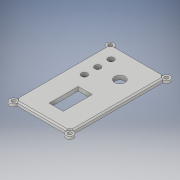
# Autodesk Inventor part: gora
Saved by Autodesk Inventor 2019 (Build 230136000, 136)
## iProperties
Created: 2019-09-16
Part Number: gora
Material: Ogólny
Document SubType Name: Modeling
Designer: mikol
Density: 1 g/cm^3
Appearance: Domyślna
Author: mikol
Autodesk Inventor part; units mm, degrees
ref_plane "YZ Plane" through (0, 0, 0) normal (1, 0, 0) x (0, 1, 0)
ref_plane "XZ Plane" through (0, 0, 0) normal (0, 1, 0) x (-1, 0, 0)
ref_plane "XY Plane" through (0, 0, 0) normal (0, 0, 1) x (1, 0, 0)
sketch "Sketch1" plane through (0, 0, 0) normal (0, 1, 0) x (-1, 0, 0)
  line L0 (32, 55) -> (-32, 55)
  line L1 (-32, 55) -> (-32, -55)
  line L2 (-32, -55) -> (32, -55)
  line L3 (32, -55) -> (32, 55)
  line L4 (32, 55) -> (-32, -55) construction
  line L5 (-32, 55) -> (32, -55) construction
  circle A0 centre (32, 55) radius 4.2425
  circle A1 centre (32, -55) radius 4.2425
  circle A2 centre (-32, 55) radius 4.2425
  circle A3 centre (-32, -55) radius 4.2425
  point P0 (0, 0)
  dimension "d0" = 64
  dimension "d1" = 110
  dimension "d2" = 8.485
  dimension "d5" = 110
  dimension "d8" = 64
  constraints: 12 end point, 4 centre point, 2 horizontal, 2 midpoint, 2 parallel, 1 coincident, 1 perpendicular, 1 vertical, 6 other
  measures "d0" distance of L2.end L1.end
  measures "d1" distance of L1.end L0.end
  measures "d2" diameter of A0
  measures "d5" distance of A0.centre A1.centre
  measures "d8" distance of A0.centre A2.centre
extrude "Extrusion1" add sketch "Sketch1" along normal blind 3
sketch "Sketch2" plane through (0, 3, 0) normal (0, 1, 0) x (1, 0, 0)
  line L0 (32, -50.7575) -> (32, 50.7575) projected
  arc A0 (32, 50.7575) -> (27.7575, 55) centre (32, 55) ccw projected
  line L1 (27.7575, 55) -> (-27.7575, 55) projected
  arc A1 (-27.7575, 55) -> (-32, 50.7575) centre (-32, 55) ccw projected
  line L2 (-32, 50.7575) -> (-32, -50.7575) projected
  arc A2 (-32, -50.7575) -> (-27.7575, -55) centre (-32, -55) ccw projected
  line L3 (-27.7575, -55) -> (27.7575, -55) projected
  arc A3 (27.7575, -55) -> (32, -50.7575) centre (32, -55) ccw projected
  circle A4 centre (-32, -55) radius 2.15
  circle A5 centre (-32, 55) radius 2.15
  circle A6 centre (32, -55) radius 2.15
  circle A7 centre (32, 55) radius 2.15
  point P0 (0, 0)
  dimension "d13" = 4.3
  dimension "d16" = 110
  dimension "d19" = 64
  constraints: 4 centre point, 1 coincident, 1 horizontal, 1 vertical, 6 other
  measures "d13" diameter of A4
  measures "d16" distance of A4.centre A5.centre
  measures "d19" distance of A4.centre A6.centre
extrude "Extrusion2" cut sketch "Sketch2" against normal blind 3 contours A4 | A5 | A6 | A7
sketch "Sketch3" plane through (0, 3, 0) normal (0, 1, 0) x (1, 0, 0)
  line L0 (-8, -38.5) -> (8, -38.5)
  line L1 (8, -38.5) -> (8, -5.5)
  line L2 (8, -5.5) -> (-8, -5.5)
  line L3 (-8, -5.5) -> (-8, -38.5)
  line L4 (-32, 50.7575) -> (-32, -50.7575) projected
  line L5 (32, -50.7575) -> (32, 50.7575) projected
  line L6 (-27.7575, -55) -> (27.7575, -55) projected
  point P0 (0, 0)
  dimension "d24" = 16
  dimension "d25" = 33
  dimension "d26" = 24
  dimension "d27" = 24
  dimension "d28" = 16.5
  constraints: 8 end point, 2 parallel, 1 horizontal, 1 perpendicular
  measures "d24" distance of L2.end L1.end
  measures "d25" distance of L1.end L0.end
  measures "d26" distance between parallel lines of L4 L3
  measures "d27" distance between parallel lines of L5 L1
  measures "d28" distance between parallel lines of L6 L0
extrude "Extrusion3" cut sketch "Sketch3" against normal blind 3
sketch "Sketch4" plane through (0, 3, 0) normal (0, 1, 0) x (1, 0, 0)
  circle A0 centre (-16, 9.625) radius 3.4
  line L0 (0, 82.9395) -> (0, -82.9395) projected
  circle A1 centre (-16, 24.75) radius 3.4
  circle A2 centre (-16, 39.875) radius 3.4
  line L1 (27.7575, 55) -> (-27.7575, 55) projected
  line L2 (-8, -5.5) -> (8, -5.5) projected
  line L3 (-16, 0) -> (-16, 55)
  circle A3 centre (9, 25) radius 6
  line L4 (32, -50.7575) -> (32, 50.7575) projected
  point P0 (0, 0)
  dimension "d31" = 6.8
  dimension "d32" = 6.8
  dimension "d33" = 6.8
  dimension "d34" = 15.125
  dimension "d35" = 15.125
  dimension "d36" = 15.125
  dimension "d37" = 15.125
  dimension "d53" = 16
  dimension "d54" = 55
  dimension "d55" = 12
  dimension "d56" = 23
  dimension "d64" = 30
  constraints: 4 centre point, 4 point on line, 2 end point, 1 vertical
  measures "d31" diameter of A0
  measures "d32" diameter of A1
  measures "d33" diameter of A2
  measures "d34" distance of A1.centre A0.centre
  measures "d35" distance of A2.centre A1.centre
  measures "d36" distance from line of L1 A2.centre
  measures "d37" distance from line of L2 A0.centre
  measures "d53" distance between parallel lines of L0 L3
  measures "d54" distance of L3.start L3.end
  measures "d55" diameter of A3
  measures "d56" distance from line of L4 A3.centre
  measures "d64" distance from line of L1 A3.centre
extrude "Extrusion4" cut sketch "Sketch4" against normal blind 6
sketch "Sketch5" plane through (0, 3, 0) normal (0, 1, 0) x (1, 0, 0)
  circle A0 centre (-16, 24.75) radius 3.4 projected
  circle A1 centre (-16, 9.625) radius 3.4 projected
  circle A2 centre (-16, 39.875) radius 3.4 projected
  line L0 (8, -5.5) -> (8, -38.5) projected
  line L1 (8, -38.5) -> (-8, -38.5) projected
  line L2 (-8, -38.5) -> (-8, -5.5) projected
  line L3 (-8, -5.5) -> (8, -5.5) projected
  circle A3 centre (32, -55) radius 2.15 projected
  circle A4 centre (-32, -55) radius 2.15 projected
  circle A5 centre (-32, 55) radius 2.15 projected
  circle A6 centre (32, 55) radius 2.15 projected
  line L4 (32, -50.7575) -> (32, 50.7575) projected
  arc A7 (32, 50.7575) -> (27.7575, 55) centre (32, 55) ccw projected
  line L5 (27.7575, 55) -> (-27.7575, 55) projected
  arc A8 (-27.7575, 55) -> (-32, 50.7575) centre (-32, 55) ccw projected
  line L6 (-32, 50.7575) -> (-32, -50.7575) projected
  arc A9 (-32, -50.7575) -> (-27.7575, -55) centre (-32, -55) ccw projected
  line L7 (-27.7575, -55) -> (27.7575, -55) projected
  arc A10 (27.7575, -55) -> (32, -50.7575) centre (32, -55) ccw projected
  circle A11 centre (-32, -55) radius 2.15 projected
  circle A12 centre (-32, -55) radius 4.2425
  circle A13 centre (-32, 55) radius 4.2425
  circle A14 centre (32, -55) radius 4.2425
  circle A15 centre (32, 55) radius 4.2425
  line L8 (-32, -50.7575) -> (-32, 50.7575)
  line L9 (-27.7575, 55) -> (27.7575, 55)
  line L10 (32, -50.7575) -> (32, 50.7575) projected
  line L11 (32, 50.7575) -> (32, -50.7575)
  line L12 (-27.7575, -55) -> (27.7575, -55) projected
  line L13 (27.7575, -55) -> (-27.7575, -55)
  circle A16 centre (-16, 39.875) radius 3.4 projected
  circle A17 centre (-16, 9.625) radius 3.4 projected
  circle A18 centre (-16, 24.75) radius 3.4 projected
  circle A19 centre (9, 25) radius 6 projected
  line L14 (8, -38.5) -> (8, -5.5) projected
  line L15 (8, -5.5) -> (-8, -5.5) projected
  line L16 (-8, -5.5) -> (-8, -38.5) projected
  line L17 (-8, -38.5) -> (8, -38.5) projected
  circle A20 centre (32, -55) radius 2.15 projected
  circle A21 centre (-32, -55) radius 2.15 projected
  circle A22 centre (-32, 55) radius 2.15 projected
  circle A23 centre (32, 55) radius 2.15 projected
  line L18 (-27.7575, -55) -> (27.7575, -55) projected
  arc A24 (-32, -50.7575) -> (-27.7575, -55) centre (-32, -55) ccw projected
  line L19 (-32, 50.7575) -> (-32, -50.7575) projected
  arc A25 (-27.7575, 55) -> (-32, 50.7575) centre (-32, 55) ccw projected
  line L20 (27.7575, 55) -> (-27.7575, 55) projected
  arc A26 (32, 50.7575) -> (27.7575, 55) centre (32, 55) ccw projected
  line L21 (32, -50.7575) -> (32, 50.7575) projected
  arc A27 (27.7575, -55) -> (32, -50.7575) centre (32, -55) ccw projected
  circle A28 centre (9, 25) radius 6
  point P0 (0, 0)
  dimension "d42" = 110
  dimension "d45" = 64
  constraints: 8 end point, 5 centre point, 3 vertical, 2 coincident, 2 collinear, 1 concentric, 1 horizontal, 9 other
  measures "d42" distance of A12.centre A13.centre
  measures "d45" distance of A12.centre A14.centre
extrude "Extrusion6" add sketch "Sketch5" along normal blind 1.5 contours A14 L7 A12 L6 A13 L5 A15 L4
chamfer "Chamfer2" distance 1.5 angle 45 4 edges at (-32, 4.5, 0) (0, 4.5, 55) (32, 4.5, 0) (0, 4.5, -55)
equation "\"d26\" = d27"
equation "\"d32\" = d31"
equation "\"d33\" = d31"
equation "\"d34\" = d37"
equation "\"d35\" = d34"
equation "\"d36\" = d34"
body "Solid1"
